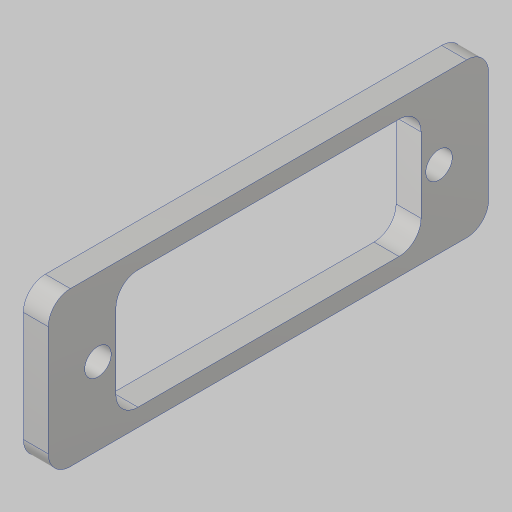
# Autodesk Inventor part: Spacer
Saved by Autodesk Inventor 2023.5 (Build 275446000, 446)
## iProperties
Created: 2025-02-08
Part Number: Spacer
Material: Aluminum 6061
Document SubType Name: Modeling
Designer: slick
Density: 2.7 g/cm^3
Appearance: Aluminum - Flat
Author: slick
Autodesk Inventor part; units mm, degrees
ref_plane "YZ Plane" through (0, 0, 0) normal (1, 0, 0) x (0, 1, 0)
ref_plane "XZ Plane" through (0, 0, 0) normal (0, 1, 0) x (-1, 0, 0)
ref_plane "XY Plane" through (0, 0, 0) normal (0, 0, 1) x (1, 0, 0)
sketch "Sketch1" plane through (0, 0, 0) normal (1, 0, 0) x (0, 1, 0)
  line L0 (-11.1125, -31.75) -> (11.1125, -31.75)
  line L1 (11.1125, -31.75) -> (11.1125, 31.75)
  line L2 (11.1125, 31.75) -> (-11.1125, 31.75)
  line L3 (-11.1125, 31.75) -> (-11.1125, -31.75)
  line L4 (-11.1125, -31.75) -> (11.1125, 31.75) construction
  line L5 (11.1125, -31.75) -> (-11.1125, 31.75) construction
  point P0 (0, 0)
  dimension "d0" = 63.5
  dimension "d1" = 22.225
  constraints: 12 end point, 2 midpoint, 2 parallel, 1 horizontal, 1 perpendicular
  measures "d0" distance of L0.end L1.end
  measures "d1" distance between parallel lines of L3 L1
extrude "Extrusion1" add sketch "Sketch1" along normal blind 3.6
sketch "Sketch2" plane through (3.6, 0, 0) normal (1, 0, 0) x (0, 0, -1)
  line L0 (22, -8.5725) -> (-22, -8.5725)
  line L1 (-22, -8.5725) -> (-22, 8.5725)
  line L2 (-22, 8.5725) -> (22, 8.5725)
  line L3 (22, 8.5725) -> (22, -8.5725)
  line L4 (22, -8.5725) -> (-22, 8.5725) construction
  line L5 (-22, -8.5725) -> (22, 8.5725) construction
  circle A0 centre (-24.5942, 0) radius 3 construction
  circle A1 centre (24.5942, 0) radius 3 construction
  line L6 (-27.5942, 0) -> (27.5942, 0) construction
  arc A2 (-25.8022, 2.746) -> (-22, 8.5725) centre (-28.3653, 8.5725) ccw
  line L7 (0, 8.5725) -> (0, -8.5725) construction
  arc A3 (-22, -8.5725) -> (-25.8022, -2.746) centre (-28.3653, -8.5725) ccw
  arc A4 (22, 8.5725) -> (25.8022, 2.746) centre (28.3653, 8.5725) ccw
  arc A5 (25.8022, -2.746) -> (22, -8.5725) centre (28.3653, -8.5725) ccw
  arc A6 (-25.8022, 2.746) -> (-25.8022, -2.746) centre (-24.5942, 0) ccw
  arc A7 (25.8022, -2.746) -> (25.8022, 2.746) centre (24.5942, 0) ccw
  point P0 (0, 0)
  point P1 (0, 0)
  dimension "d4" = 44
  dimension "d5" = 17.145
  dimension "d7" = 6
  dimension "d20" = 49.1884
  constraints: 16 end point, 14 point on circle, 7 centre point, 6 coincident, 6 symmetric about line, 5 midpoint, 3 horizontal alignment, 2 horizontal, 2 parallel, 2 tangent, 1 perpendicular, 1 point on line, 6 other
  measures "d4" distance of L1.end L2.end
  measures "d5" distance of L0.end L1.end
  measures "d7" diameter of A0
  measures "d20" distance of A7.centre A0.centre
extrude "Extrusion2" cut sketch "Sketch2" against normal blind 3.6 contours L0 L1 L2 L3
hole "Hole1" at (3.6, 0, 24.5942) at (3.6, 0, -24.5942) direction (-1, 0, 0) diameter 3.81 end through all clearance for "Flat Head Machine Screw (82)" size "#6" standard "Ansi Unified Screw Threads"
fillet "Fillet1" radius 3.175 8 edges at (1.8, 8.5725, 22) (1.8, 11.1125, 31.75) (1.8, -11.1125, 31.75) (1.8, -8.5725, 22) (1.8, -8.5725, -22) (1.8, -11.1125, -31.75) (1.8, 11.1125, -31.75) (1.8, 8.5725, -22)
body "Solid1"
